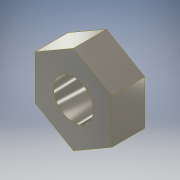
# Autodesk Inventor part: Porca M3
Saved by Autodesk Inventor 2018 (Build 220112000, 112)
## iProperties
Created: 2017-09-07
Part Number: Porca M3
Material: Genérico
Document SubType Name: Modeling
Designer: caeta
Density: 1 g/cm^3
Appearance: Prata
Author: caeta
Autodesk Inventor part; units mm, degrees
ref_plane "YZ Plane" through (0, 0, 0) normal (1, 0, 0) x (0, 1, 0)
ref_plane "XZ Plane" through (0, 0, 0) normal (0, 1, 0) x (-1, 0, 0)
ref_plane "XY Plane" through (0, 0, 0) normal (0, 0, 1) x (1, 0, 0)
sketch "Esboço1" plane through (0, 0, 0) normal (0, 1, 0) x (-1, 0, 0)
  line L0 (0, -4.5815) -> (-2.9062, -6.2522)
  line L1 (-2.9062, -6.2522) -> (-5.8062, -4.5707)
  line L2 (-5.8062, -4.5707) -> (-5.8, -1.2185)
  line L3 (-5.8, -1.2185) -> (-2.8938, 0.4522)
  line L4 (-2.8938, 0.4522) -> (0.0062, -1.2293)
  line L5 (0.0062, -1.2293) -> (0, -4.5815)
  circle A0 centre (-2.9, -2.9) radius 1.5
  point P0 (0, 0)
  dimension "d11" = 3
  constraints: 12 end point, 1 centre point, 1 coincident, 13 other
  measures "d11" diameter of A0
extrude "Extrusão1" add sketch "Esboço1" along normal blind 2.5
